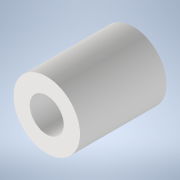
# Autodesk Inventor part: StangePotiAdapter1
Saved by Autodesk Inventor 2020.3 (Build 243373010, 373A)
## iProperties
Created: 2020-11-30
Part Number: StangePotiAdapter1
Material: Generisch
Document SubType Name: Modeling
Designer: Stefan
Density: 1 g/cm^3
Appearance: Vorgabe
Author: Stefan
Autodesk Inventor part; units mm, degrees
ref_plane "YZ Plane" through (0, 0, 0) normal (1, 0, 0) x (0, 1, 0)
ref_plane "XZ Plane" through (0, 0, 0) normal (0, 1, 0) x (-1, 0, 0)
ref_plane "XY Plane" through (0, 0, 0) normal (0, 0, 1) x (1, 0, 0)
sketch "Skizze1" plane through (0, 0, 0) normal (0, 0, 1) x (1, 0, 0)
  circle A0 centre (0, 0) radius 10
  circle A1 centre (0, 0) radius 5.1
  line L0 (0, 0) -> (0, 25.1367) construction
  dimension "d0" = 20
  dimension "d1" = 10.2
  constraints: 3 coincident, 2 centre point, 2 end point, 1 vertical
  measures "d0" diameter of A0
  measures "d1" diameter of A1
extrude "Extrusion1" add sketch "Skizze1" along normal blind 16
sketch "Skizze2" plane through (0, 0, 0) normal (0, 0, -1) x (-1, 0, 0)
  circle A0 centre (0, 0) radius 10
  line L0 (5.05, 2.55) -> (-5.05, 2.55)
  line L1 (-5.05, 2.55) -> (-5.05, -2.55)
  line L2 (-5.05, -2.55) -> (5.05, -2.55)
  line L3 (5.05, -2.55) -> (5.05, 2.55)
  dimension "d9" = 20
  dimension "d10" = 10.1
  dimension "d11" = 5.1
  dimension "d12" = 5.05
  dimension "d13" = 2.55
  constraints: 8 end point, 2 parallel, 1 centre point, 1 coincident, 1 horizontal, 1 perpendicular
  measures "d9" diameter of A0
  measures "d10" distance of L2.end L1.end
  measures "d11" distance of L1.end L0.end
  measures "d12" distance from line of point (0, 0) L3
  measures "d13" distance from line of point (0, 0) L2
extrude "Extrusion2" add sketch "Skizze2" along normal blind 10
